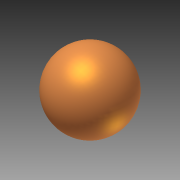
# Autodesk Inventor part: BasketBall
Saved by Autodesk Inventor 2012 (Build 160160000, 160)
## iProperties
Created: 2012-10-25
Part Number: BasketBall
Material: Rubber
Document SubType Name: Modeling
Designer: Andrew G. Meyer
Mass: 514.608 g
Surface Area: 3486.04 cm^2
Volume: 553.342 cm^3
Density: 0.93 g/cm^3
Author: Andrew G. Meyer
Autodesk Inventor part; units mm, degrees
ref_plane "YZ Plane" through (0, 0, 0) normal (1, 0, 0) x (0, 1, 0)
ref_plane "XZ Plane" through (0, 0, 0) normal (0, 1, 0) x (-1, 0, 0)
ref_plane "XY Plane" through (0, 0, 0) normal (0, 0, 1) x (1, 0, 0)
sketch "Sketch1" plane through (0, 0, 0) normal (0, 0, 1) x (1, 0, 0)
  arc A0 (116.175, 0) -> (-116.175, 0) centre (0, 0) ccw
  arc A1 (119.35, 0) -> (-119.35, 0) centre (0, 0) ccw
  line L0 (-119.35, 0) -> (119.35, 0) construction
  line L1 (-119.35, 0) -> (-116.175, 0)
  line L2 (119.35, 0) -> (116.175, 0)
  dimension "d0" = 238.7
  dimension "d1" = 3.175
  constraints: 6 end point, 4 point on circle, 2 centre point, 2 coincident, 2 collinear, 2 point on line, 1 horizontal, 1 midpoint
  measures "d0" diameter of A1
  measures "d1" radial gap between concentric circles of A0 A1
revolve "Revolution1" add sketch "Sketch1" angle 360 about axis through (-119.35, 0, 0) along (1, 0, 0)
body "Solid1"
